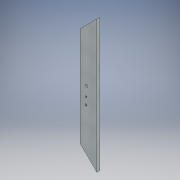
# Autodesk Inventor part: Fata_4
Saved by Autodesk Inventor 2017 (Build 210142000, 142)
## iProperties
Created: 2017-06-02
Part Number: Fata_4
Material: Generic
Document SubType Name: Modeling
Designer: crush
Density: 1 g/cm^3
Appearance: Wood - Painted White
Author: crush
Autodesk Inventor part; units mm, degrees
ref_plane "YZ Plane" through (0, 0, 0) normal (1, 0, 0) x (0, 1, 0)
ref_plane "XZ Plane" through (0, 0, 0) normal (0, 1, 0) x (-1, 0, 0)
ref_plane "XY Plane" through (0, 0, 0) normal (0, 0, 1) x (1, 0, 0)
sketch "Sketch1" plane through (0, 0, 0) normal (0, 1, 0) x (-1, 0, 0)
  line L0 (0, 0) -> (0, -600)
  line L1 (0, 0) -> (-100, 0)
  line L2 (-100, 0) -> (-100, 100)
  line L3 (-100, 100) -> (0, 0)
  line L4 (0, -600) -> (-100, -600)
  line L5 (-100, -600) -> (-100, -700)
  line L6 (-100, -700) -> (0, -600)
  line L7 (-100, -600) -> (-100, 0)
  dimension "d0" = 600
  dimension "d1" = 100
  dimension "d2" = 100
  dimension "d3" = 100
  dimension "d4" = 100
  constraints: 16 end point, 2 horizontal, 2 perpendicular, 2 vertical
  measures "d0" distance of L0.start L0.end
  measures "d1" distance of L0.start L1.end
  measures "d2" distance of L1.end L2.end
  measures "d3" distance of L0.end L4.end
  measures "d4" distance of L4.end L5.end
extrude "Extrusion1" add sketch "Sketch1" along normal blind 18
sketch "Sketch3" plane through (0, 18, 0) normal (0, 1, 0) x (1, 0, 0)
  circle A0 centre (38.9698, 279.3172) radius 7.5
  line L0 (100, 700) -> (0, 600)
  line L1 (0, 0) -> (100, -100)
  line L2 (0, 0) -> (100, -100) projected
  line L3 (100, -100) -> (100, 700) projected
  line L4 (100, 700) -> (0, 600) projected
  line L5 (0, 600) -> (0, 0) projected
  constraints: 4 end point, 1 centre point
extrude "Extrusion2" cut sketch "Sketch3" against normal blind 20 contours A0
sketch "Sketch4" plane through (0, 0, 0) normal (0, -1, 0) x (1, 0, 0)
  circle A0 centre (38.9698, -279.3172) radius 7.5
  line L0 (100, 100) -> (100, -700)
  line L1 (17.2005, -615) -> (17.2005, 25)
  line L2 (22.2005, -326.9779) -> (47.2005, -326.9779)
  line L3 (47.2005, -326.9779) -> (47.2005, -391.9779)
  line L4 (47.2005, -391.9779) -> (22.2005, -391.9779)
  line L5 (0, -600) -> (0, 0)
  line L6 (100, -700) -> (0, -600)
  line L7 (0, 0) -> (100, 100)
  circle A1 centre (38.9698, -279.3539) radius 7.5
  circle A2 centre (38.9698, -279.3539) radius 4.625
  circle A3 centre (38.9698, -279.3539) radius 5.75
  circle A4 centre (38.7754, -333.8918) radius 1
  circle A5 centre (34.7754, -333.8918) radius 1
  circle A6 centre (30.7754, -333.8918) radius 1
  circle A7 centre (38.7754, -337.8918) radius 1
  circle A8 centre (34.7754, -337.8918) radius 1
  circle A9 centre (30.7754, -337.8918) radius 1
  circle A10 centre (38.7754, -341.8918) radius 1
  circle A11 centre (34.7754, -341.8918) radius 1
  circle A12 centre (30.7754, -341.8918) radius 1
  circle A13 centre (38.7005, -377.1197) radius 1
  circle A14 centre (34.7005, -377.1197) radius 1
  circle A15 centre (30.7005, -377.1197) radius 1
  circle A16 centre (38.7005, -381.1197) radius 1
  circle A17 centre (34.7005, -381.1197) radius 1
  circle A18 centre (30.7005, -381.1197) radius 1
  circle A19 centre (38.7005, -385.1197) radius 1
  circle A20 centre (34.7005, -385.1197) radius 1
  circle A21 centre (30.7005, -385.1197) radius 1
  dimension "d9" = 2
  dimension "d12" = 4
  dimension "d15" = 4
  dimension "d18" = 2
  dimension "d19" = 4
  dimension "d20" = 4
  constraints: 22 centre point, 16 end point, 1 horizontal, 1 vertical
  measures "d9" diameter of A4
  measures "d12" distance of A4.centre A5.centre
  measures "d15" distance of A4.centre A7.centre
  measures "d18" diameter of A13
  measures "d19" distance of A13.centre A14.centre
  measures "d20" distance of A13.centre A16.centre
extrude "Extrusion3" cut sketch "Sketch4" against normal blind 20 contours A4 | A5 | A6 | A7 | A8 | A9 | A10 | A11 | A12 | A13 | A14 | A15 | A16 | A17 | A18 | A19 | A20 | A21
body "Solid1"
